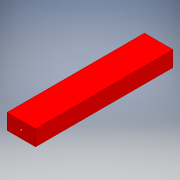
# Autodesk Inventor part: Battery_small
Saved by Autodesk Inventor 2018 (Build 220112000, 112)
## iProperties
Created: 2017-12-31
Part Number: Battery_small
Material: Generic
Document SubType Name: Modeling
Designer: suchanek
Density: 1 g/cm^3
Appearance: Default
Mass: 3.498 g
Surface Area: 19.34 cm^2
Volume: 3.498 cm^3
Author: suchanek
Autodesk Inventor part; units mm, degrees
ref_plane "YZ Plane" through (0, 0, 0) normal (1, 0, 0) x (0, 1, 0)
ref_plane "XZ Plane" through (0, 0, 0) normal (0, 1, 0) x (-1, 0, 0)
ref_plane "XY Plane" through (0, 0, 0) normal (0, 0, 1) x (1, 0, 0)
sketch "Sketch1" plane through (0, 0, 0) normal (0, 1, 0) x (-1, 0, 0)
  point P0 (0, 0)
sketch "Sketch2" plane through (0, 0, 0) normal (0, 1, 0) x (-1, 0, 0)
  line L0 (0, 0) -> (5.5, 0)
  line L1 (5.5, 0) -> (5.5, 3)
  line L2 (5.5, 3) -> (0, 3)
  line L3 (0, 3) -> (0, 0)
  line L4 (5.5, 3) -> (-5.5, 3)
  line L5 (-5.5, 3) -> (-5.5, -3)
  line L6 (-5.5, -3) -> (5.5, -3)
  line L7 (5.5, -3) -> (5.5, 3)
  dimension "d0" = 5.5
  dimension "d1" = 3
  dimension "d2" = 11
  dimension "d3" = 6
  constraints: 16 end point, 4 parallel, 2 horizontal, 2 perpendicular
  measures "d0" distance of L2.end L1.end
  measures "d1" distance of L1.end L0.end
  measures "d2" distance of L6.end L5.end
  measures "d3" distance of L5.end L4.end
extrude "Extrusion1" add sketch "Sketch2" along normal blind 53
body "Solid1"
